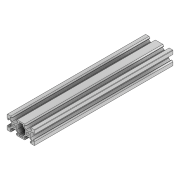
# Autodesk Inventor part: Perfil2040
Saved by Autodesk Inventor 2021 (Build 250183000, 183)
## iProperties
Created: 2021-02-12
Part Number: Perfil2040
Material: Aluminio 6061
Document SubType Name: Modeling
Designer: sddj_
Density: 2.7 g/cm^3
Appearance: Aluminio - Pulido
Author: sddj_
Autodesk Inventor part; units mm, degrees
ref_plane "YZ Plane" through (0, 0, 0) normal (1, 0, 0) x (0, 1, 0)
ref_plane "XZ Plane" through (0, 0, 0) normal (0, 1, 0) x (-1, 0, 0)
ref_plane "XY Plane" through (0, 0, 0) normal (0, 0, 1) x (1, 0, 0)
sketch "Boceto1" plane through (0, 0, 0) normal (0, 0, 1) x (1, 0, 0)
  circle A0 centre (0, 0) radius 2.1
  line L0 (-12, 0) -> (12, 0)
  line L1 (0, 12) -> (0, -12)
  line L2 (0, 3.9) -> (-2.8387, 3.9)
  line L3 (-2.8387, 3.9) -> (-5.5, 6.555)
  line L4 (-5.5, 6.555) -> (-5.5, 8.195)
  line L5 (-5.5, 8.195) -> (-3.125, 8.195)
  line L6 (-3.125, 8.545) -> (-4.58, 10)
  line L7 (-4.58, 10) -> (-10, 10)
  line L8 (-10, 10) -> (-10, 4.58)
  line L9 (-10, 4.58) -> (-8.5415, 3.125)
  line L10 (-8.1915, 3.125) -> (-8.1915, 5.4852)
  line L11 (-8.1915, 5.4852) -> (-6.5515, 5.4852)
  line L12 (-6.5515, 5.4852) -> (-3.9, 2.84)
  line L13 (-3.9, 2.84) -> (-3.9, 0)
  line L14 (3.125, 8.545) -> (4.58, 10)
  line L15 (5.5, 8.195) -> (3.125, 8.195)
  line L16 (5.5, 6.555) -> (5.5, 8.195)
  line L17 (2.8387, 3.9) -> (5.5, 6.555)
  line L18 (0, 3.9) -> (2.8387, 3.9)
  line L19 (3.9, 2.84) -> (3.9, 0)
  line L20 (-10, -10) -> (-10, -4.58)
  line L21 (-4.58, -10) -> (-10, -10)
  line L22 (-3.125, -8.545) -> (-4.58, -10)
  line L23 (-5.5, -8.195) -> (-3.125, -8.195)
  line L24 (-5.5, -6.555) -> (-5.5, -8.195)
  line L25 (-2.8387, -3.9) -> (-5.5, -6.555)
  line L26 (0, -3.9) -> (-2.8387, -3.9)
  line L27 (0, -3.9) -> (2.8387, -3.9)
  line L28 (2.8387, -3.9) -> (5.5, -6.555)
  line L29 (5.5, -6.555) -> (5.5, -8.195)
  line L30 (5.5, -8.195) -> (3.125, -8.195)
  line L31 (3.125, -8.545) -> (4.58, -10)
  line L32 (7.3, -6.2319) -> (3.9, -2.84)
  line L33 (3.9, -2.84) -> (3.9, 0)
  line L34 (-3.9, -2.84) -> (-3.9, 0)
  line L35 (-6.5515, -5.4852) -> (-3.9, -2.84)
  line L36 (-8.1915, -5.4852) -> (-6.5515, -5.4852)
  line L37 (-8.1915, -3.125) -> (-8.1915, -5.4852)
  line L38 (-10, -4.58) -> (-8.5415, -3.125)
  line L39 (-3.125, 8.195) -> (-3.125, 8.545)
  line L40 (-8.1915, 3.125) -> (-8.5415, 3.125)
  line L41 (3.125, 8.195) -> (3.125, 8.545)
  line L42 (-8.1915, -3.125) -> (-8.5415, -3.125)
  line L43 (-3.125, -8.195) -> (-3.125, -8.545)
  line L44 (3.125, -8.195) -> (3.125, -8.545)
  line L45 (10, 12) -> (10, -12)
  line L46 (16.875, 8.195) -> (16.875, 8.545)
  line L47 (14.5, 8.195) -> (16.875, 8.195)
  line L48 (14.5, 6.555) -> (14.5, 8.195)
  line L49 (16.875, 8.545) -> (15.42, 10)
  line L50 (17.1613, 3.9) -> (14.5, 6.555)
  line L51 (20, 3.9) -> (17.1613, 3.9)
  line L52 (32, 0) -> (8, 0)
  line L53 (20, 3.9) -> (22.8387, 3.9)
  line L54 (23.125, 8.195) -> (23.125, 8.545)
  circle A1 centre (20, 0) radius 2.1
  line L55 (23.9, -2.84) -> (23.9, 0)
  line L56 (26.5515, -5.4852) -> (23.9, -2.84)
  line L57 (28.1915, -5.4852) -> (26.5515, -5.4852)
  line L58 (24.58, -10) -> (30, -10)
  line L59 (30, -10) -> (30, -4.58)
  line L60 (28.1915, -3.125) -> (28.1915, -5.4852)
  line L61 (30, -4.58) -> (28.5415, -3.125)
  line L62 (28.1915, -3.125) -> (28.5415, -3.125)
  line L63 (22.8387, -3.9) -> (25.5, -6.555)
  line L64 (25.5, -8.195) -> (23.125, -8.195)
  line L65 (23.125, -8.195) -> (23.125, -8.545)
  line L66 (23.125, -8.545) -> (24.58, -10)
  line L67 (20, -3.9) -> (22.8387, -3.9)
  line L68 (20, -3.9) -> (17.1613, -3.9)
  line L69 (16.875, -8.195) -> (16.875, -8.545)
  line L70 (25.5, -6.555) -> (25.5, -8.195)
  line L71 (12.7, -6.2319) -> (16.1, -2.84)
  line L72 (17.1613, -3.9) -> (14.5, -6.555)
  line L73 (14.5, -8.195) -> (16.875, -8.195)
  line L74 (16.875, -8.545) -> (15.42, -10)
  line L75 (14.5, -6.555) -> (14.5, -8.195)
  line L76 (20, 12) -> (20, -12)
  line L77 (22.8387, 3.9) -> (25.5, 6.555)
  line L78 (25.5, 6.555) -> (25.5, 8.195)
  line L79 (25.5, 8.195) -> (23.125, 8.195)
  line L80 (23.125, 8.545) -> (24.58, 10)
  line L81 (24.58, 10) -> (30, 10)
  line L82 (30, 10) -> (30, 4.58)
  line L83 (30, 4.58) -> (28.5415, 3.125)
  line L84 (28.1915, 3.125) -> (28.1915, 5.4852)
  line L85 (28.1915, 5.4852) -> (26.5515, 5.4852)
  line L86 (26.5515, 5.4852) -> (23.9, 2.84)
  line L87 (23.9, 2.84) -> (23.9, 0)
  line L88 (28.1915, 3.125) -> (28.5415, 3.125)
  line L89 (16.1, 2.84) -> (16.1, 0)
  line L90 (16.1, -2.84) -> (16.1, 0)
  line L91 (7.3, -6.2319) -> (7.3, -8.195)
  line L92 (7.3, -8.195) -> (12.7, -8.195)
  line L93 (12.7, -8.195) -> (12.7, -6.2319)
  line L94 (4.58, 10) -> (15.42, 10)
  line L95 (4.58, -10) -> (15.42, -10)
  line L96 (3.9, 2.84) -> (7.3, 6.2319)
  line L97 (7.3, 6.2319) -> (7.3, 8.195)
  line L98 (7.3, 8.195) -> (12.7, 8.195)
  line L99 (12.7, 8.195) -> (12.7, 6.2319)
  line L100 (16.1, 2.84) -> (12.7, 6.2319)
  point P0 (10, 0)
  dimension "d0" = 4.2
  dimension "d1" = 24
  dimension "d2" = 24
  dimension "d3" = 90
  dimension "d6" = 20
  dimension "d7" = 1.5
  dimension "d8" = 1.64
  dimension "d9" = 1.64
  dimension "d10" = 7.8
  dimension "d11" = 11
  dimension "d12" = 9.16
  dimension "d14" = 6.25
  dimension "d15" = 6.25
  dimension "d16" = 0.35
  dimension "d17" = 7.8
  dimension "d18" = 0.35
  dimension "d20" = 24
  dimension "d24" = 12.2
  dimension "d25" = 9.16
  dimension "d26" = 5.68
  dimension "d31" = 5.4
  dimension "d32" = 5.4
  dimension "d34" = 40
  constraints: 202 end point, 83 symmetric about line, 9 perpendicular, 8 parallel, 7 coincident, 5 midpoint, 5 vertical, 4 point on line, 3 collinear, 3 horizontal, 2 centre point, 2 horizontal alignment, 1 other
  measures "d0" diameter of A0
  measures "d1" distance of L0.start L0.end
  measures "d2" distance of L1.start L1.end
  measures "d3" angle of L14 L6
  measures "d6" distance of L21.end L7.end
  measures "d7" distance between parallel lines of L3 L12
  measures "d8" distance of L3.end L4.end
  measures "d9" distance of L10.end L11.end
  measures "d10" distance between parallel lines of L19 L13
  measures "d11" distance between parallel lines of L16 L4
  measures "d12" distance of L14.end L6.end
  measures "d14" distance between parallel lines of L41 L39
  measures "d15" distance between parallel lines of L42 L40
  measures "d16" distance of L10.start L9.end
  measures "d17" distance between parallel lines of L26 L2
  measures "d18" distance of L39.start L39.end
  measures "d20" distance of L45.start L45.end
  measures "d24" distance between parallel lines of L89 L19
  measures "d25" distance of L8.end L20.end
  measures "d26" distance of L32.end L19.start
  measures "d31" distance between parallel lines of L99 L97
  measures "d32" distance between parallel lines of L93 L91
  measures "d34" distance between parallel lines of L59 L20
extrude "Extrusión1" add sketch "Boceto1" against normal blind 200 contours L0 L33 L32 L91 L92 L45 L95 L31 L44 L30 L29 L28 L27 L1 A0 | A0 L1 L18 L17 L16 L15 L41 L14 L94 L45 L98 L97 L96 L19 L0 | A0 L0 L13 L12 L11 L10 L40 L9 L8 L7 L6 L39 L5 L4 L3 L2 L1 | L1 L26 L25 L24 L23 L43 L22 L21 L20 L38 L42 L37 L36 L35 L34 L0 A0 | L45 L94 L49 L46 L47 L48 L50 L51 L76 A1 L52 L89 L100 L99 L98 | L92 L93 L71 L90 L52 A1 L76 L68 L72 L75 L73 L69 L74 L95 L45 | L76 L53 L77 L78 L79 L54 L80 L81 L82 L83 L88 L84 L85 L86 L87 L52 A1 | A1 L52 L55 L56 L57 L60 L62 L61 L59 L58 L66 L65 L64 L70 L63 L67 L76
fillet "Empalme1" radius 0.5 4 edges at (-10, 10, -100) (30, 10, -100) (30, -10, -100) (-10, -10, -100)
